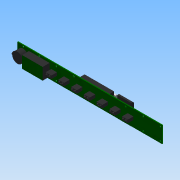
# Autodesk Inventor part: electronics
Saved by Autodesk Inventor 2015 (Build 190159000, 159)
## iProperties
Created: 2015-08-10
Part Number: electronics
Material: Générique
Document SubType Name: Modeling
Designer: Gregwar
Density: 1 g/cm^3
Appearance: Par défaut
Author: Gregwar
Autodesk Inventor part; units mm, degrees
ref_plane "YZ Plane" through (0, 0, 0) normal (1, 0, 0) x (0, 1, 0)
ref_plane "XZ Plane" through (0, 0, 0) normal (0, 1, 0) x (-1, 0, 0)
ref_plane "XY Plane" through (0, 0, 0) normal (0, 0, 1) x (1, 0, 0)
sketch "Esquisse1" plane through (0, 0, 0) normal (0, 1, 0) x (-1, 0, 0)
  line L0 (0, 0) -> (250, 0)
  line L1 (250, 0) -> (250, -28)
  line L2 (250, -28) -> (0, -28)
  line L3 (0, -28) -> (0, 0)
  dimension "d0" = 250
  dimension "d1" = 28
  constraints: 8 end point, 2 parallel, 1 horizontal, 1 perpendicular
  measures "d0" distance of L0.start L0.end
  measures "d1" distance of L2.end L0.start
extrude "Extrusion1" add sketch "Esquisse1" along normal blind 1.6
sketch "Esquisse2" plane through (0, 1.6, 0) normal (0, 1, 0) x (1, 0, 0)
  circle A0 centre (-3, 3) radius 1.5
  line L0 (0, 0) -> (0, 28) construction
  line L1 (0, 14) -> (-250, 14) construction
  line L2 (-250, 28) -> (-250, 0) construction
  line L3 (-250, 0) -> (0, 0) construction
  circle A1 centre (-33, 3) radius 1.5
  circle A2 centre (-63, 3) radius 1.5
  circle A3 centre (-153, 3) radius 1.5
  circle A4 centre (-183, 3) radius 1.5
  circle A5 centre (-213, 3) radius 1.5
  circle A6 centre (-3, 25) radius 1.5
  circle A7 centre (-33, 25) radius 1.5
  circle A8 centre (-63, 25) radius 1.5
  circle A9 centre (-153, 25) radius 1.5
  circle A10 centre (-183, 25) radius 1.5
  circle A11 centre (-213, 25) radius 1.5
  line L4 (-240, 0) -> (-240, 28) construction
  line L5 (0, 28) -> (-250, 28) construction
  circle A12 centre (-240, 2.3) radius 1.5
  circle A13 centre (-240, 25.7) radius 1.5
  dimension "d4" = 3
  dimension "d5" = 3
  dimension "d6" = 3
  dimension "d9" = 30
  dimension "d16" = 90
  dimension "d23" = 30
  dimension "d28" = 2.3
  dimension "d29" = 3
  dimension "d30" = 10
  constraints: 14 centre point, 7 symmetric about line, 4 end point, 3 horizontal, 3 point on line, 2 midpoint, 1 vertical, 17 other
  measures "d4" diameter of A0
  measures "d5" distance from line of L3 A0.centre
  measures "d6" distance from line of L0 A0.centre
  measures "d9" distance of A0.centre A1.centre
  measures "d16" distance of A2.centre A3.centre
  measures "d23" distance of A3.centre A4.centre
  measures "d28" distance from line of L3 A12.centre
  measures "d29" diameter of A12
  measures "d30" distance between parallel lines of L4 L2
extrude "Extrusion2" cut sketch "Esquisse2" against normal through all
sketch "Esquisse3" plane through (0, 0, 0) normal (0, -1, 0) x (1, 0, 0)
  line L0 (0, -28) -> (0, 0) construction
  line L1 (0, -14) -> (-250, -14) construction
  line L2 (-250, 0) -> (-250, -28) construction
  line L3 (-181.5, -11.35) -> (-191.5, -11.35)
  line L4 (-191.5, -11.35) -> (-191.5, -16.65)
  line L5 (-191.5, -16.65) -> (-181.5, -16.65)
  line L6 (-181.5, -16.65) -> (-181.5, -11.35)
  line L7 (-181.5, -14) -> (-191.5, -14) construction
  dimension "d33" = 5.3
  dimension "d34" = 10
  dimension "d35" = 58.5
  constraints: 12 end point, 4 midpoint, 2 parallel, 1 collinear, 1 horizontal, 1 perpendicular
  measures "d33" distance of L3.end L4.end
  measures "d34" distance of L4.end L5.end
  measures "d35" distance between parallel lines of L2 L4
extrude "Extrusion3" add sketch "Esquisse3" along normal blind 9.8
sketch "Esquisse4" plane through (0, -9.8, 0) normal (0, -1, 0) x (1, 0, 0)
  line L0 (-181.5, -11.35) -> (-191.5, -11.35) construction
  line L1 (-191.5, -11.35) -> (-191.5, -16.65) construction
  line L2 (-191.5, -16.65) -> (-181.5, -16.65) construction
  line L3 (-181.5, -16.65) -> (-181.5, -11.35) construction
  line L4 (-191.5, -11.35) -> (-181.5, -11.35) construction
  line L5 (-186.5, -11.35) -> (-186.5, -16.65) construction
  line L6 (-186.5, -14) -> (-181.5, -14) construction
  circle A0 centre (-184, -14) radius 2
  line L7 (-182, -14) -> (-186, -14) construction
  line L8 (-182, -14) -> (-186, -14)
  line L9 (-191.5, -16.65) -> (-181.5, -16.65) projected
  line L10 (-186.5, -14) -> (-191.5, -14) construction
  circle A1 centre (-189, -14) radius 2
  line L11 (-191, -14) -> (-187, -14)
  point P0 (0, 0)
  dimension "d61" = 4
  constraints: 12 end point, 5 midpoint, 4 symmetric about line, 2 centre point, 2 point on circle, 2 point on line, 1 parallel, 1 other
  measures "d61" diameter of A0
revolve "Révolution1" add sketch "Esquisse4" angle 360 about axis through (-186.5, -9.8, -14) along (-1, 0, 0) picked at (-184.499, -14.7612) contours A0 L8
ref_plane "Plan de construction1" through (-186.5, 0, -16.65) normal (-1, 0, 0) x (0, 0, 1)
mirror "Symétrie1" about plane through (-186.5, 0, -16.65) normal (-1, 0, 0) of "Révolution1"
pattern_linear "Réseau rectangulaire1" count 7 spacing 22 along (1, 0, 0) of "Extrusion3", "Révolution1", "Symétrie1"
sketch "Esquisse8" plane through (0, 1.6, 0) normal (0, 1, 0) x (1, 0, 0)
  line L0 (-97, 4.75) -> (-148, 4.75)
  line L1 (-148, 4.75) -> (-148, 23.25)
  line L2 (-148, 23.25) -> (-97, 23.25)
  line L3 (-97, 23.25) -> (-97, 4.75)
  line L4 (-250, 0) -> (-250, 28) construction
  line L5 (-250, 14) -> (0, 14) construction
  line L6 (-97, 14) -> (-148, 14) construction
  line L7 (0, 0) -> (0, 28) construction
  dimension "d51" = 51
  dimension "d52" = 18.5
  dimension "d53" = 97
  constraints: 12 end point, 3 midpoint, 2 horizontal, 2 parallel, 1 collinear, 1 perpendicular
  measures "d51" distance of L0.start L0.end
  measures "d52" distance of L0.end L1.end
  measures "d53" distance between parallel lines of L3 L7
extrude "Extrusion6" add sketch "Esquisse8" along normal blind 12.5
sketch "Esquisse9" plane through (0, 14.1, 0) normal (0, 1, 0) x (1, 0, 0)
  line L0 (-95, 10.1) -> (-104.3, 10.1)
  line L1 (-104.3, 10.1) -> (-104.3, 17.9)
  line L2 (-104.3, 17.9) -> (-95, 17.9)
  line L3 (-95, 17.9) -> (-95, 10.1)
  line L4 (-104.3, 14) -> (-95, 14) construction
  line L5 (-148, 23.25) -> (-148, 4.75) construction
  line L6 (-148, 14) -> (-97, 14) construction
  line L7 (-97, 4.75) -> (-97, 23.25) construction
  point P0 (0, 0)
  dimension "d57" = 9.3
  dimension "d58" = 7.8
  dimension "d80" = 2
  constraints: 12 end point, 4 midpoint, 2 parallel, 1 collinear, 1 horizontal, 1 perpendicular
  measures "d57" distance between parallel lines of L3 L1
  measures "d58" distance of L2.end L0.start
  measures "d80" distance between parallel lines of L7 L3
extrude "Extrusion7" add sketch "Esquisse9" along normal blind 3.8
ref_plane "Plan de construction2" through (0, 0.8, 0) normal (0, 1, 0) x (1, 0, 0)
sketch "Esquisse12" plane through (0, 0, 0) normal (0, -1, 0) x (1, 0, 0)
  circle A0 centre (-240, -25.7) radius 1.5 construction
  line L0 (-240, -2.3) -> (-240, -25.7) construction
  circle A1 centre (-240, -14) radius 9
  circle A2 centre (-240, -2.3) radius 1.5 construction
  point P0 (0, 0)
  dimension "d66" = 18
  constraints: 2 end point, 1 centre point, 1 coincident, 1 midpoint, 1 vertical
  measures "d66" diameter of A1
extrude "Extrusion9" add sketch "Esquisse12" along normal blind 9.8
sketch "Esquisse13" plane through (-250, 0, -28) normal (-1, 0, 0) x (0, 0, 1)
  circle A0 centre (10, -2.2) radius 2.5
  line L0 (0, 0) -> (0, 1.6) projected
  line L1 (0, 1.6) -> (28, 1.6) projected
  point P0 (28, 0)
  dimension "d69" = 5
  dimension "d70" = 10
  dimension "d71" = 3.8
  constraints: 1 centre point
  measures "d69" diameter of A0
  measures "d70" distance from line of L0 A0.centre
  measures "d71" distance from line of L1 A0.centre
extrude "Extrusion10" add sketch "Esquisse13" along normal mid plane 10
chamfer "Chanfrein2" distance 1 angle 45 2 edges at (-99.65, 17.9, -17.9) (-99.65, 17.9, -10.1)
shell "Coque2" thickness 0.5 removed faces 1 at (-95, 15.3667, -13.0333)
sketch "Esquisse15" plane through (-103.8, 13.6, -10.6) normal (1, 0, 0) x (0, 0, -1)
  line L0 (0.7071, 3.8) -> (0, 3.0929) projected
  line L1 (0, 0) -> (0, 3.0929) projected
  line L2 (0, 0) -> (6.8, 0) projected
  line L3 (6.8, 0) -> (6.8, 3.0929) projected
  line L4 (6.8, 3.0929) -> (6.0929, 3.8) projected
  line L5 (6.0929, 3.8) -> (0.7071, 3.8) projected
  point P0 (-10.6, -13.6)
extrude "Extrusion12" add sketch "Esquisse15" along normal blind 7
sketch "Esquisse18" plane through (0, 1.6, 0) normal (0, 1, 0) x (1, 0, 0)
  circle A0 centre (-189, 14) radius 2 construction
  circle A1 centre (-184, 14) radius 2 construction
  line L0 (-181.5, 11.35) -> (-191.5, 11.35) construction
  line L1 (-191.5, 11.35) -> (-191.5, 16.65) construction
  line L2 (-191.5, 16.65) -> (-181.5, 16.65) construction
  line L3 (-181.5, 16.65) -> (-181.5, 11.35) construction
  circle A2 centre (-167, 14) radius 2 construction
  circle A3 centre (-162, 14) radius 2 construction
  line L4 (-159.5, 11.35) -> (-169.5, 11.35) construction
  line L5 (-169.5, 11.35) -> (-169.5, 16.65) construction
  line L6 (-169.5, 16.65) -> (-159.5, 16.65) construction
  line L7 (-159.5, 16.65) -> (-159.5, 11.35) construction
  line L8 (-169.5, 14) -> (-181.5, 14) construction
  line L9 (-180.5, 11.35) -> (-170.5, 11.35)
  line L10 (-170.5, 11.35) -> (-170.5, 16.65)
  line L11 (-170.5, 16.65) -> (-180.5, 16.65)
  line L12 (-180.5, 16.65) -> (-180.5, 11.35)
  line L13 (-180.5, 14) -> (-170.5, 14) construction
  point P0 (0, 0)
  point P1 (-175.5, 14)
  constraints: 12 end point, 6 midpoint, 2 equal length, 2 parallel, 1 horizontal, 1 perpendicular
extrude "Extrusion14" add sketch "Esquisse18" along normal blind 9.8
sketch "Esquisse19" plane through (0, 11.4, 0) normal (0, 1, 0) x (1, 0, 0)
  line L0 (-180.5, 11.35) -> (-170.5, 11.35) construction
  line L1 (-170.5, 11.35) -> (-170.5, 16.65) construction
  line L2 (-170.5, 16.65) -> (-180.5, 16.65) construction
  line L3 (-180.5, 16.65) -> (-180.5, 11.35) construction
  line L4 (-175.5, 11.35) -> (-175.5, 16.65) construction
  line L5 (-175.5, 14) -> (-180.5, 14) construction
  circle A0 centre (-178, 14) radius 2
  line L6 (-176, 14) -> (-180, 14)
  point P0 (0, 0)
  dimension "d93" = 4
  constraints: 6 end point, 5 midpoint, 2 point on circle, 2 point on line, 1 centre point
  measures "d93" diameter of A0
revolve "Révolution4" add sketch "Esquisse19" angle 360 about axis through (-175.5, 11.4, -14) along (-1, 0, 0) picked at (-177.501, 14.7612) contours L6 A0
ref_plane "Plan de construction5" through (-175.5, 1.6, -16.65) normal (-1, 0, 0) x (0, 0, 1)
mirror "Symétrie4" about plane through (-175.5, 1.6, -16.65) normal (-1, 0, 0) of "Révolution4"
sketch "Esquisse20" plane through (0, 1.6, 0) normal (0, 1, 0) x (1, 0, 0)
  line L0 (-55, -5.2) -> (-79, -5.2)
  line L1 (-79, -5.2) -> (-79, 29.8)
  line L2 (-79, 29.8) -> (-55, 29.8)
  line L3 (-55, 29.8) -> (-55, -5.2)
  line L4 (-97, 4.75) -> (-97, 10.1) projected
  line L5 (-250, 0) -> (0, 0) projected
  dimension "d95" = 18
  dimension "d96" = 24
  dimension "d97" = 35
  dimension "d98" = 5.2
  constraints: 8 end point, 2 parallel, 1 horizontal, 1 perpendicular
  measures "d95" distance between parallel lines of L1 L4
  measures "d96" distance of L0.start L0.end
  measures "d97" distance of L2.end L0.start
  measures "d98" distance between parallel lines of L5 L0
extrude "Extrusion15" add sketch "Esquisse20" along normal blind 5
chamfer "Chanfrein3" distance 2 angle 45 1 edges at (-67, 6.6, 5.2)
sketch "Esquisse21" plane through (0, 0, 0) normal (0, -1, 0) x (1, 0, 0)
  line L0 (-230, -3.75) -> (-194.3, -3.75)
  line L1 (-194.3, -3.75) -> (-194.3, -24.25)
  line L2 (-194.3, -24.25) -> (-230, -24.25)
  line L3 (-230, -24.25) -> (-230, -3.75)
  line L4 (-250, -16.8126) -> (-248.5492, -16.8126) construction
  arc A0 (-247.3546, -19.1874) -> (-248.5492, -16.8126) centre (-240, -14) ccw construction
  line L5 (-247.3546, -19.1874) -> (-250, -19.1874) construction
  line L6 (-250, -19.1874) -> (-250, -28) construction
  line L7 (-250, -28) -> (0, -28) construction
  line L8 (0, -28) -> (0, 0) construction
  line L9 (0, 0) -> (-250, 0) construction
  line L10 (-250, 0) -> (-250, -16.8126) construction
  line L11 (-49.5, -11.35) -> (-49.5, -16.65) construction
  line L12 (-49.5, -16.65) -> (-59.5, -16.65) construction
  line L13 (-59.5, -16.65) -> (-59.5, -11.35) construction
  line L14 (-59.5, -11.35) -> (-49.5, -11.35) construction
  line L15 (-71.5, -11.35) -> (-71.5, -16.65) construction
  line L16 (-71.5, -16.65) -> (-81.5, -16.65) construction
  line L17 (-81.5, -16.65) -> (-81.5, -11.35) construction
  line L18 (-81.5, -11.35) -> (-71.5, -11.35) construction
  line L19 (-93.5, -11.35) -> (-93.5, -16.65) construction
  line L20 (-93.5, -16.65) -> (-103.5, -16.65) construction
  line L21 (-103.5, -16.65) -> (-103.5, -11.35) construction
  line L22 (-103.5, -11.35) -> (-93.5, -11.35) construction
  line L23 (-115.5, -11.35) -> (-115.5, -16.65) construction
  line L24 (-115.5, -16.65) -> (-125.5, -16.65) construction
  line L25 (-125.5, -16.65) -> (-125.5, -11.35) construction
  line L26 (-125.5, -11.35) -> (-115.5, -11.35) construction
  line L27 (-137.5, -11.35) -> (-137.5, -16.65) construction
  line L28 (-137.5, -16.65) -> (-147.5, -16.65) construction
  line L29 (-147.5, -16.65) -> (-147.5, -11.35) construction
  line L30 (-147.5, -11.35) -> (-137.5, -11.35) construction
  line L31 (-159.5, -11.35) -> (-159.5, -16.65) construction
  line L32 (-159.5, -16.65) -> (-169.5, -16.65) construction
  line L33 (-169.5, -16.65) -> (-169.5, -11.35) construction
  line L34 (-169.5, -11.35) -> (-159.5, -11.35) construction
  line L35 (-181.5, -11.35) -> (-181.5, -16.65) construction
  line L36 (-181.5, -16.65) -> (-191.5, -16.65) construction
  line L37 (-191.5, -16.65) -> (-191.5, -11.35) construction
  line L38 (-191.5, -11.35) -> (-181.5, -11.35) construction
  circle A1 centre (-240, -2.3) radius 1.5 construction
  circle A2 centre (-183, -25) radius 1.5 construction
  circle A3 centre (-63, -25) radius 1.5 construction
  circle A4 centre (-3, -25) radius 1.5 construction
  circle A5 centre (-183, -3) radius 1.5 construction
  circle A6 centre (-63, -3) radius 1.5 construction
  circle A7 centre (-3, -3) radius 1.5 construction
  circle A8 centre (-33, -3) radius 1.5 construction
  circle A9 centre (-153, -3) radius 1.5 construction
  circle A10 centre (-213, -3) radius 1.5 construction
  circle A11 centre (-33, -25) radius 1.5 construction
  circle A12 centre (-153, -25) radius 1.5 construction
  circle A13 centre (-213, -25) radius 1.5 construction
  circle A14 centre (-240, -25.7) radius 1.5 construction
  line L39 (-249.5, -0.5) -> (-249.5, -27.5) construction
  line L40 (-249.5, -14) -> (-191.5, -14) construction
  line L41 (-191.5, -16.65) -> (-191.5, -11.35) construction
  line L42 (-230, -14) -> (-194.3, -14) construction
  dimension "d104" = 35.7
  dimension "d105" = 20.5
  dimension "d106" = 20
  constraints: 12 end point, 4 midpoint, 2 parallel, 1 collinear, 1 horizontal, 1 perpendicular
  measures "d104" distance of L0.start L0.end
  measures "d105" distance of L0.end L1.end
  measures "d106" distance between parallel lines of L10 L3
extrude "Extrusion16" add sketch "Esquisse21" along normal blind 12
